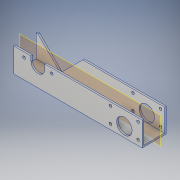
# Autodesk Inventor part: CAR_042_KickerLBracket
Saved by Autodesk Inventor 2018.3 (Build 223284000, 284)
## iProperties
Created: 2020-02-13
Part Number: CAR_042_KickerLBracket
Material: Aluminum 6061
Document SubType Name: Modeling
Designer: user
Mass: 257.174 g
Surface Area: 625.604 cm^2
Volume: 95.2498 cm^3
Density: 2.7 g/cm^3
Appearance: Aluminum - Flat
Author: user
Autodesk Inventor part; units mm, degrees
ref_plane "YZ Plane" through (0, 0, 0) normal (1, 0, 0) x (0, 1, 0)
ref_plane "XZ Plane" through (0, 0, 0) normal (0, 1, 0) x (-1, 0, 0)
ref_plane "XY Plane" through (0, 0, 0) normal (0, 0, 1) x (1, 0, 0)
sketch "Sketch1" plane through (0, 0, 0) normal (1, 0, 0) x (0, 1, 0)
  line L0 (41.275, -22.225) -> (-3.175, -22.225)
  line L1 (-3.175, -22.225) -> (-3.175, 22.225)
  line L2 (-3.175, 22.225) -> (41.275, 22.225)
  line L3 (0, 19.05) -> (0, -19.05)
  line L4 (0, 19.05) -> (41.275, 19.05)
  line L5 (0, -19.05) -> (41.275, -19.05)
  line L6 (41.275, 22.225) -> (41.275, 19.05)
  line L7 (41.275, -19.05) -> (41.275, -22.225)
  point P0 (0, 0)
  point P1 (0, 0)
  dimension "d27" = 44.45
  dimension "d28" = 44.45
  dimension "d29" = 3.175
  dimension "d83" = 3.175
  constraints: 16 end point, 3 horizontal, 3 parallel, 2 equal length, 1 coincident, 1 midpoint, 1 perpendicular
  measures "d27" distance of L1.end L2.end
  measures "d28" distance of L0.end L1.end
  measures "d29" distance between parallel lines of L1 L3
  measures "d83" distance between parallel lines of L4 L2
extrude "Extrusion1" add sketch "Sketch1" along normal blind 236.1946
sketch "Sketch4" plane through (0, -3.175, -22.225) normal (0, 0, -1) x (-1, 0, 0)
  line L0 (0, 3.175) -> (0, 0) projected
  line L1 (-44.45, 101.8817) -> (-44.45, -23.3371)
  line L2 (0, 3.175) -> (-236.1946, 3.175) projected
  point P0 (-19.05, 35.56)
  point P1 (-69.85, 35.56)
  dimension "d30" = 50.8
  dimension "d81" = 25.4
  dimension "d82" = 44.45
  dimension "d84" = 32.385
  constraints: 2 end point, 1 horizontal alignment, 1 vertical
  measures "d30" distance of point (-69.85, 35.56) point (-19.05, 35.56)
  measures "d81" distance from line of point (-19.05, 35.56) L1
  measures "d82" distance between parallel lines of L1 L0
  measures "d84" distance from line of L2 point (-19.05, 35.56)
hole "Hole2" at (19.05, 32.385, -22.225) at (69.85, 32.385, -22.225) direction (0, 0, 1) diameter 5.1054 end through all clearance for "Flat Head Machine Screw (82)" size "#10" standard "Ansi Unified Screw Threads"
sketch "Sketch7" plane through (0, -3.175, 0) normal (0, 0, 1) x (1, 0, 0)
  line L0 (-1.0792, 48.7042) -> (44.45, 94.2334)
  line L1 (44.45, 94.2334) -> (89.9792, 48.7042)
  line L2 (89.9792, 48.7042) -> (44.45, 3.175)
  line L3 (44.45, 3.175) -> (-1.0792, 48.7042)
  line L4 (0, 0) -> (0, 44.45) projected
  line L5 (0, 0) -> (236.1946, 0) projected
  line L6 (44.45, 3.175) -> (44.45, -64.4339)
  circle A0 centre (19.05, 35.56) radius 2.5527 projected
  circle A1 centre (69.85, 35.56) radius 2.5527 projected
  point P0 (0, 3.175)
  dimension "d57" = 3.175
  dimension "d85" = 50.8
  dimension "d86" = 25.4
  dimension "d87" = 135
  constraints: 10 end point, 2 parallel, 1 perpendicular, 1 vertical, 1 vertical alignment
  measures "d57" distance from line of L5 L2.end
  measures "d85" distance of A1.centre A0.centre
  measures "d86" distance from line of A0.centre L6
  measures "d87" angle of L6 L3
extrude "Extrusion3" cut sketch "Sketch7" against normal through all contours L0 L1 L2 L3 | A0 | A1
sketch "Sketch10" plane through (0, -3.175, 0) normal (0, 0, 1) x (1, 0, 0)
  line L0 (31.75, 54.9704) -> (57.15, 54.9704)
  line L1 (57.15, 54.9704) -> (57.15, 35.56)
  line L2 (31.75, 35.56) -> (31.75, 54.9704)
  arc A0 (31.75, 35.56) -> (57.15, 35.56) centre (44.45, 35.56) ccw
  circle A1 centre (19.05, 35.56) radius 2.5527 projected
  point P0 (0, 3.175)
  point P1 (44.45, 3.175)
  dimension "d88" = 25.4
  constraints: 6 end point, 2 point on circle, 2 tangent, 1 centre point, 1 horizontal, 1 horizontal alignment, 1 parallel, 1 perpendicular, 1 vertical alignment
  measures "d88" distance of L0.start L0.end
extrude "Extrusion5" cut sketch "Sketch10" along normal through all contours L0 L1 A0 L2
sketch "Sketch11" plane through (0, -3.175, -22.225) normal (0, 0, -1) x (-1, 0, 0)
  line L0 (-236.1946, 0) -> (-236.1946, 44.45) projected
  line L1 (0, 0) -> (-236.1946, 0) projected
  arc A0 (-57.15, 35.56) -> (-31.75, 35.56) centre (-44.45, 35.56) ccw projected
  line L2 (-85.725, 44.45) -> (-236.1946, 44.45) projected
  point P0 (0, 3.175)
  point P1 (-203.537, 18.542)
  point P2 (-236.1946, 22.225)
  dimension "d89" = 159.9946
  dimension "d114" = 25.908
  constraints: 1 coincident, 1 midpoint
  measures "d89" distance of point (-203.537, 18.542) point (-44.45, 35.56)
  measures "d114" distance from line of point (-203.537, 18.542) L2
hole "Hole5" at (203.537, 15.367, -22.225) direction (0, 0, 1) diameter 28.5496 end through all
sketch "Sketch12" plane through (0, -3.175, -22.225) normal (0, 0, -1) x (-1, 0, 0)
  circle A0 centre (-203.537, 18.542) radius 14.2748 projected
  line L0 (0, 0) -> (-236.1946, 0) projected
  point P0 (0, 3.175)
  point P1 (-178.137, 38.1)
  point P2 (-178.137, 9.525)
  point P3 (-228.937, 9.525)
  point P4 (-228.937, 38.1)
  dimension "d99" = 9.525
  dimension "d100" = 38.1
  dimension "d101" = 25.4
  dimension "d102" = 25.4
  constraints: 2 horizontal alignment, 2 vertical alignment
  measures "d99" distance from line of point (-228.937, 9.525) L0
  measures "d100" distance from line of point (-228.937, 38.1) L0
  measures "d101" horizontal distance of point (-228.937, 9.525) A0.centre
  measures "d102" horizontal distance of point (-178.137, 9.525) A0.centre
hole "Hole6" at (178.137, 34.925, -22.225) at (178.137, 6.35, -22.225) at (228.937, 6.35, -22.225) at (228.937, 34.925, -22.225) direction (0, 0, 1) diameter 5.1054 end through all clearance for "Flat Head Machine Screw (82)" size "#10" standard "Ansi Unified Screw Threads"
sketch "Sketch8" plane through (0, 0, 19.05) normal (0, 1, 0) x (1, 0, 0)
  line L0 (64.7446, 19.05) -> (90.1446, 19.05) construction
  line L1 (64.7446, 15.494) -> (90.1446, 15.494)
  line L2 (90.1446, 22.606) -> (64.7446, 22.606)
  arc A0 (64.7446, 22.606) -> (64.7446, 15.494) centre (64.7446, 19.05) ccw
  arc A1 (90.1446, 15.494) -> (90.1446, 22.606) centre (90.1446, 19.05) ccw
  line L3 (115.5446, 19.05) -> (140.9446, 19.05) construction
  line L4 (115.5446, 15.494) -> (140.9446, 15.494)
  line L5 (140.9446, 22.606) -> (115.5446, 22.606)
  arc A2 (115.5446, 22.606) -> (115.5446, 15.494) centre (115.5446, 19.05) ccw
  arc A3 (140.9446, 15.494) -> (140.9446, 22.606) centre (140.9446, 19.05) ccw
  line L6 (236.1946, 38.1) -> (236.1946, 0) projected
  line L7 (0, 0) -> (0, 38.1) projected
  point P0 (77.4446, 19.05)
  point P1 (128.2446, 19.05)
  point P2 (0, 19.05)
  dimension "d62" = 25.4
  dimension "d64" = 107.95
  dimension "d80" = 158.75
  dimension "d115" = 7.112
  constraints: 16 end point, 8 point on circle, 8 tangent, 4 centre point, 3 midpoint, 2 horizontal, 2 parallel, 2 point on line, 1 collinear, 1 equal radius
  measures "d62" distance of L2.start L2.end
  measures "d64" distance from line of point (128.245, 19.05) L6
  measures "d80" distance from line of point (77.445, 19.05) L6
  measures "d115" diameter of A1
extrude "Extrusion4" cut sketch "Sketch8" against normal through all
ref_plane "Work Plane1" through (0, -3.175, 0) normal (0, 0, 1) x (1, 0, 0)
sketch "Sketch2" plane through (0, 0, 0) normal (0, 0, 1) x (1, 0, 0)
  circle A0 centre (23.8125, 23.8125) radius 25.4
  line L0 (5.852, 64.6197) -> (5.852, -28.4292) construction
  line L1 (0, 50.8) -> (0, 0) construction
  line L2 (0, 0) -> (304.8, 0) construction
  line L3 (304.8, 50.8) -> (304.8, 0) construction
  line L4 (0, 50.8) -> (304.8, 50.8) construction
  line L5 (0, 47.625) -> (304.8, 47.625) construction
  point P0 (5.852, 5.852)
  point P1 (41.773, 5.852)
  point P2 (41.773, 41.773)
  point P3 (5.852, 41.773)
  dimension "d11" = 50.8
  dimension "d14" = 360
  dimension "d16" = 5.852
  dimension "d17" = 5.852
  dimension "d19" = 5.852
  constraints: 2 end point, 2 point on line, 1 vertical, 8 other
  measures "d16" distance from line of L5 point (5.852, 41.773)
  measures "d17" distance from line of L2 point (5.852, 5.852)
  measures "d19" distance between parallel lines of L0 L1
equation "\"d83\" = d29"
equation "\"d81\" = 0.5 * d30"
equation "\"d86\" = 0.5 * d85"
equation "\"d16\" = d17"
equation "\"d19\" = d17"
body "Solid1"
